Autodesk Inventor part; units mm, degrees
(part 2 of 2)
sketch "Sketch2" plane through (2, 0, 0) normal (1, 0, 0) x (0, 0, -1)
  line L0 (27.4898, 96.0981) -> (27.4898, 576.0981) projected
  line L1 (27.4898, 576.0981) -> (-362.5102, 576.0981) projected
  line L2 (-362.5102, 576.0981) -> (-362.5102, 96.0981) projected
  line L3 (-362.5102, 96.0981) -> (27.4898, 96.0981) projected
  circle A0 centre (-37.5102, 103.5981) radius 1.75 projected
  circle A1 centre (-297.5102, 568.5981) radius 1.75 projected
  circle A2 centre (-37.5102, 568.5981) radius 1.75 projected
  circle A3 centre (-355.0102, 161.0981) radius 1.75 projected
  circle A4 centre (-355.0102, 511.0981) radius 1.75 projected
  circle A5 centre (19.9898, 161.0981) radius 1.75 projected
  circle A6 centre (19.9898, 511.0981) radius 1.75 projected
  circle A7 centre (-167.5102, 568.5981) radius 1.75 projected
  circle A8 centre (-297.5102, 103.5981) radius 1.75 projected
  line L4 (7.265, 163.0981) -> (1.4915, 163.0981) projected
  line L5 (1.4915, 163.0981) -> (-1.3952, 168.0981) projected
  line L6 (-1.3952, 168.0981) -> (1.4915, 173.0981) projected
  line L7 (1.4915, 173.0981) -> (7.265, 173.0981) projected
  line L8 (7.265, 173.0981) -> (10.1518, 168.0981) projected
  line L9 (10.1518, 168.0981) -> (7.265, 163.0981) projected
  line L10 (-18.735, 143.0981) -> (-15.8482, 138.0981) projected
  line L11 (-15.8482, 138.0981) -> (-18.735, 133.0981) projected
  line L12 (-18.735, 133.0981) -> (-24.5085, 133.0981) projected
  line L13 (-24.5085, 133.0981) -> (-27.3952, 138.0981) projected
  line L14 (-27.3952, 138.0981) -> (-24.5085, 143.0981) projected
  line L15 (-24.5085, 143.0981) -> (-18.735, 143.0981) projected
  line L16 (-40.3856, 160.5981) -> (-37.4988, 165.5981) projected
  line L17 (-37.4988, 165.5981) -> (-31.7253, 165.5981) projected
  line L18 (-31.7253, 165.5981) -> (-28.8386, 160.5981) projected
  line L19 (-28.8386, 160.5981) -> (-31.7253, 155.5981) projected
  line L20 (-31.7253, 155.5981) -> (-37.4988, 155.5981) projected
  line L21 (-37.4988, 155.5981) -> (-40.3856, 160.5981) projected
  line L22 (-50.5085, 128.0981) -> (-44.735, 128.0981) projected
  line L23 (-44.735, 128.0981) -> (-41.8482, 123.0981) projected
  line L24 (-41.8482, 123.0981) -> (-44.735, 118.0981) projected
  line L25 (-44.735, 118.0981) -> (-50.5085, 118.0981) projected
  line L26 (-50.5085, 118.0981) -> (-53.3952, 123.0981) projected
  line L27 (-53.3952, 123.0981) -> (-50.5085, 128.0981) projected
  line L28 (-67.8482, 168.0981) -> (-70.735, 163.0981) projected
  line L29 (-70.735, 163.0981) -> (-76.5085, 163.0981) projected
  line L30 (-76.5085, 163.0981) -> (-79.3952, 168.0981) projected
  line L31 (-79.3952, 168.0981) -> (-76.5085, 173.0981) projected
  line L32 (-76.5085, 173.0981) -> (-70.735, 173.0981) projected
  line L33 (-70.735, 173.0981) -> (-67.8482, 168.0981) projected
  line L34 (-92.3856, 130.5981) -> (-89.4988, 135.5981) projected
  line L35 (-89.4988, 135.5981) -> (-83.7253, 135.5981) projected
  line L36 (-83.7253, 135.5981) -> (-80.8386, 130.5981) projected
  line L37 (-80.8386, 130.5981) -> (-83.7253, 125.5981) projected
  line L38 (-83.7253, 125.5981) -> (-89.4988, 125.5981) projected
  line L39 (-89.4988, 125.5981) -> (-92.3856, 130.5981) projected
  line L40 (-102.5085, 158.0981) -> (-96.735, 158.0981) projected
  line L41 (-96.735, 158.0981) -> (-93.8482, 153.0981) projected
  line L42 (-93.8482, 153.0981) -> (-96.735, 148.0981) projected
  line L43 (-96.735, 148.0981) -> (-102.5085, 148.0981) projected
  line L44 (-102.5085, 148.0981) -> (-105.3952, 153.0981) projected
  line L45 (-105.3952, 153.0981) -> (-102.5085, 158.0981) projected
  line L46 (-115.4988, 140.5981) -> (-118.3856, 145.5981) projected
  line L47 (-118.3856, 145.5981) -> (-115.4988, 150.5981) projected
  line L48 (-115.4988, 150.5981) -> (-109.7253, 150.5981) projected
  line L49 (-109.7253, 150.5981) -> (-106.8386, 145.5981) projected
  line L50 (-106.8386, 145.5981) -> (-109.7253, 140.5981) projected
  line L51 (-109.7253, 140.5981) -> (-115.4988, 140.5981) projected
  line L52 (-122.735, 143.0981) -> (-119.8482, 138.0981) projected
  line L53 (-119.8482, 138.0981) -> (-122.735, 133.0981) projected
  line L54 (-122.735, 133.0981) -> (-128.5085, 133.0981) projected
  line L55 (-128.5085, 133.0981) -> (-131.3952, 138.0981) projected
  line L56 (-131.3952, 138.0981) -> (-128.5085, 143.0981) projected
  line L57 (-128.5085, 143.0981) -> (-122.735, 143.0981) projected
  line L58 (-148.735, 143.0981) -> (-145.8482, 138.0981) projected
  line L59 (-145.8482, 138.0981) -> (-148.735, 133.0981) projected
  line L60 (-148.735, 133.0981) -> (-154.5085, 133.0981) projected
  line L61 (-154.5085, 133.0981) -> (-157.3952, 138.0981) projected
  line L62 (-157.3952, 138.0981) -> (-154.5085, 143.0981) projected
  line L63 (-154.5085, 143.0981) -> (-148.735, 143.0981) projected
  line L64 (-154.5085, 158.0981) -> (-148.735, 158.0981) projected
  line L65 (-148.735, 158.0981) -> (-145.8482, 153.0981) projected
  line L66 (-145.8482, 153.0981) -> (-148.735, 148.0981) projected
  line L67 (-148.735, 148.0981) -> (-154.5085, 148.0981) projected
  line L68 (-154.5085, 148.0981) -> (-157.3952, 153.0981) projected
  line L69 (-157.3952, 153.0981) -> (-154.5085, 158.0981) projected
  line L70 (-171.8482, 168.0981) -> (-174.735, 163.0981) projected
  line L71 (-174.735, 163.0981) -> (-180.5085, 163.0981) projected
  line L72 (-180.5085, 163.0981) -> (-183.3952, 168.0981) projected
  line L73 (-183.3952, 168.0981) -> (-180.5085, 173.0981) projected
  line L74 (-180.5085, 173.0981) -> (-174.735, 173.0981) projected
  line L75 (-174.735, 173.0981) -> (-171.8482, 168.0981) projected
  line L76 (-196.3856, 130.5981) -> (-193.4988, 135.5981) projected
  line L77 (-193.4988, 135.5981) -> (-187.7253, 135.5981) projected
  line L78 (-187.7253, 135.5981) -> (-184.8386, 130.5981) projected
  line L79 (-184.8386, 130.5981) -> (-187.7253, 125.5981) projected
  line L80 (-187.7253, 125.5981) -> (-193.4988, 125.5981) projected
  line L81 (-193.4988, 125.5981) -> (-196.3856, 130.5981) projected
  line L82 (-206.5085, 158.0981) -> (-200.735, 158.0981) projected
  line L83 (-200.735, 158.0981) -> (-197.8482, 153.0981) projected
  line L84 (-197.8482, 153.0981) -> (-200.735, 148.0981) projected
  line L85 (-200.735, 148.0981) -> (-206.5085, 148.0981) projected
  line L86 (-206.5085, 148.0981) -> (-209.3952, 153.0981) projected
  line L87 (-209.3952, 153.0981) -> (-206.5085, 158.0981) projected
  line L88 (-219.4988, 140.5981) -> (-222.3856, 145.5981) projected
  line L89 (-222.3856, 145.5981) -> (-219.4988, 150.5981) projected
  line L90 (-219.4988, 150.5981) -> (-213.7253, 150.5981) projected
  line L91 (-213.7253, 150.5981) -> (-210.8386, 145.5981) projected
  line L92 (-210.8386, 145.5981) -> (-213.7253, 140.5981) projected
  line L93 (-213.7253, 140.5981) -> (-219.4988, 140.5981) projected
  line L94 (-226.735, 143.0981) -> (-223.8482, 138.0981) projected
  line L95 (-223.8482, 138.0981) -> (-226.735, 133.0981) projected
  line L96 (-226.735, 133.0981) -> (-232.5085, 133.0981) projected
  line L97 (-232.5085, 133.0981) -> (-235.3952, 138.0981) projected
  line L98 (-235.3952, 138.0981) -> (-232.5085, 143.0981) projected
  line L99 (-232.5085, 143.0981) -> (-226.735, 143.0981) projected
  line L100 (-248.3856, 160.5981) -> (-245.4988, 165.5981) projected
  line L101 (-245.4988, 165.5981) -> (-239.7253, 165.5981) projected
  line L102 (-239.7253, 165.5981) -> (-236.8386, 160.5981) projected
  line L103 (-236.8386, 160.5981) -> (-239.7253, 155.5981) projected
  line L104 (-239.7253, 155.5981) -> (-245.4988, 155.5981) projected
  line L105 (-245.4988, 155.5981) -> (-248.3856, 160.5981) projected
  line L106 (-258.5085, 128.0981) -> (-252.735, 128.0981) projected
  line L107 (-252.735, 128.0981) -> (-249.8482, 123.0981) projected
  line L108 (-249.8482, 123.0981) -> (-252.735, 118.0981) projected
  line L109 (-252.735, 118.0981) -> (-258.5085, 118.0981) projected
  line L110 (-258.5085, 118.0981) -> (-261.3952, 123.0981) projected
  line L111 (-261.3952, 123.0981) -> (-258.5085, 128.0981) projected
  line L112 (-310.5085, 128.0981) -> (-304.735, 128.0981) projected
  line L113 (-304.735, 128.0981) -> (-301.8482, 123.0981) projected
  line L114 (-301.8482, 123.0981) -> (-304.735, 118.0981) projected
  line L115 (-304.735, 118.0981) -> (-310.5085, 118.0981) projected
  line L116 (-310.5085, 118.0981) -> (-313.3952, 123.0981) projected
  line L117 (-313.3952, 123.0981) -> (-310.5085, 128.0981) projected
  line L118 (-336.5085, 158.0981) -> (-330.735, 158.0981) projected
  line L119 (-330.735, 158.0981) -> (-327.8482, 153.0981) projected
  line L120 (-327.8482, 153.0981) -> (-330.735, 148.0981) projected
  line L121 (-330.735, 148.0981) -> (-336.5085, 148.0981) projected
  line L122 (-336.5085, 148.0981) -> (-339.3952, 153.0981) projected
  line L123 (-339.3952, 153.0981) -> (-336.5085, 158.0981) projected
  line L124 (-275.8482, 168.0981) -> (-278.735, 163.0981) projected
  line L125 (-278.735, 163.0981) -> (-284.5085, 163.0981) projected
  line L126 (-284.5085, 163.0981) -> (-287.3952, 168.0981) projected
  line L127 (-287.3952, 168.0981) -> (-284.5085, 173.0981) projected
  line L128 (-284.5085, 173.0981) -> (-278.735, 173.0981) projected
  line L129 (-278.735, 173.0981) -> (-275.8482, 168.0981) projected
  line L130 (-278.735, 143.0981) -> (-275.8482, 138.0981) projected
  line L131 (-275.8482, 138.0981) -> (-278.735, 133.0981) projected
  line L132 (-278.735, 133.0981) -> (-284.5085, 133.0981) projected
  line L133 (-284.5085, 133.0981) -> (-287.3952, 138.0981) projected
  line L134 (-287.3952, 138.0981) -> (-284.5085, 143.0981) projected
  line L135 (-284.5085, 143.0981) -> (-278.735, 143.0981) projected
  line L136 (-304.735, 143.0981) -> (-301.8482, 138.0981) projected
  line L137 (-301.8482, 138.0981) -> (-304.735, 133.0981) projected
  line L138 (-304.735, 133.0981) -> (-310.5085, 133.0981) projected
  line L139 (-310.5085, 133.0981) -> (-313.3952, 138.0981) projected
  line L140 (-313.3952, 138.0981) -> (-310.5085, 143.0981) projected
  line L141 (-310.5085, 143.0981) -> (-304.735, 143.0981) projected
  line L142 (1.4915, 128.0981) -> (7.265, 128.0981) projected
  line L143 (7.265, 128.0981) -> (10.1518, 123.0981) projected
  line L144 (10.1518, 123.0981) -> (7.265, 118.0981) projected
  line L145 (7.265, 118.0981) -> (1.4915, 118.0981) projected
  line L146 (1.4915, 118.0981) -> (-1.3952, 123.0981) projected
  line L147 (-1.3952, 123.0981) -> (1.4915, 128.0981) projected
  line L148 (-5.7253, 140.5981) -> (-11.4988, 140.5981) projected
  line L149 (-11.4988, 140.5981) -> (-14.3856, 145.5981) projected
  line L150 (-14.3856, 145.5981) -> (-11.4988, 150.5981) projected
  line L151 (-11.4988, 150.5981) -> (-5.7253, 150.5981) projected
  line L152 (-5.7253, 150.5981) -> (-2.8386, 145.5981) projected
  line L153 (-2.8386, 145.5981) -> (-5.7253, 140.5981) projected
  line L154 (-323.4988, 140.5981) -> (-326.3856, 145.5981) projected
  line L155 (-326.3856, 145.5981) -> (-323.4988, 150.5981) projected
  line L156 (-323.4988, 150.5981) -> (-317.7253, 150.5981) projected
  line L157 (-317.7253, 150.5981) -> (-314.8386, 145.5981) projected
  line L158 (-314.8386, 145.5981) -> (-317.7253, 140.5981) projected
  line L159 (-317.7253, 140.5981) -> (-323.4988, 140.5981) projected
  line L160 (-297.4988, 140.5981) -> (-300.3856, 145.5981) projected
  line L161 (-300.3856, 145.5981) -> (-297.4988, 150.5981) projected
  line L162 (-297.4988, 150.5981) -> (-291.7253, 150.5981) projected
  line L163 (-291.7253, 150.5981) -> (-288.8386, 145.5981) projected
  line L164 (-288.8386, 145.5981) -> (-291.7253, 140.5981) projected
  line L165 (-291.7253, 140.5981) -> (-297.4988, 140.5981) projected
  line L166 (-274.3856, 160.5981) -> (-271.4988, 165.5981) projected
  line L167 (-271.4988, 165.5981) -> (-265.7253, 165.5981) projected
  line L168 (-265.7253, 165.5981) -> (-262.8386, 160.5981) projected
  line L169 (-262.8386, 160.5981) -> (-265.7253, 155.5981) projected
  line L170 (-265.7253, 155.5981) -> (-271.4988, 155.5981) projected
  line L171 (-271.4988, 155.5981) -> (-274.3856, 160.5981) projected
  line L172 (-327.8482, 168.0981) -> (-330.735, 163.0981) projected
  line L173 (-330.735, 163.0981) -> (-336.5085, 163.0981) projected
  line L174 (-336.5085, 163.0981) -> (-339.3952, 168.0981) projected
  line L175 (-339.3952, 168.0981) -> (-336.5085, 173.0981) projected
  line L176 (-336.5085, 173.0981) -> (-330.735, 173.0981) projected
  line L177 (-330.735, 173.0981) -> (-327.8482, 168.0981) projected
  line L178 (-326.3856, 130.5981) -> (-323.4988, 135.5981) projected
  line L179 (-323.4988, 135.5981) -> (-317.7253, 135.5981) projected
  line L180 (-317.7253, 135.5981) -> (-314.8386, 130.5981) projected
  line L181 (-314.8386, 130.5981) -> (-317.7253, 125.5981) projected
  line L182 (-317.7253, 125.5981) -> (-323.4988, 125.5981) projected
  line L183 (-323.4988, 125.5981) -> (-326.3856, 130.5981) projected
  line L184 (-274.3856, 130.5981) -> (-271.4988, 135.5981) projected
  line L185 (-271.4988, 135.5981) -> (-265.7253, 135.5981) projected
  line L186 (-265.7253, 135.5981) -> (-262.8386, 130.5981) projected
  line L187 (-262.8386, 130.5981) -> (-265.7253, 125.5981) projected
  line L188 (-265.7253, 125.5981) -> (-271.4988, 125.5981) projected
  line L189 (-271.4988, 125.5981) -> (-274.3856, 130.5981) projected
  line L190 (-249.8482, 168.0981) -> (-252.735, 163.0981) projected
  line L191 (-252.735, 163.0981) -> (-258.5085, 163.0981) projected
  line L192 (-258.5085, 163.0981) -> (-261.3952, 168.0981) projected
  line L193 (-261.3952, 168.0981) -> (-258.5085, 173.0981) projected
  line L194 (-258.5085, 173.0981) -> (-252.735, 173.0981) projected
  line L195 (-252.735, 173.0981) -> (-249.8482, 168.0981) projected
  line L196 (-232.5085, 128.0981) -> (-226.735, 128.0981) projected
  line L197 (-226.735, 128.0981) -> (-223.8482, 123.0981) projected
  line L198 (-223.8482, 123.0981) -> (-226.735, 118.0981) projected
  line L199 (-226.735, 118.0981) -> (-232.5085, 118.0981) projected
  line L200 (-232.5085, 118.0981) -> (-235.3952, 123.0981) projected
  line L201 (-235.3952, 123.0981) -> (-232.5085, 128.0981) projected
  line L202 (-222.3856, 160.5981) -> (-219.4988, 165.5981) projected
  line L203 (-219.4988, 165.5981) -> (-213.7253, 165.5981) projected
  line L204 (-213.7253, 165.5981) -> (-210.8386, 160.5981) projected
  line L205 (-210.8386, 160.5981) -> (-213.7253, 155.5981) projected
  line L206 (-213.7253, 155.5981) -> (-219.4988, 155.5981) projected
  line L207 (-219.4988, 155.5981) -> (-222.3856, 160.5981) projected
  line L208 (-200.735, 143.0981) -> (-197.8482, 138.0981) projected
  line L209 (-197.8482, 138.0981) -> (-200.735, 133.0981) projected
  line L210 (-200.735, 133.0981) -> (-206.5085, 133.0981) projected
  line L211 (-206.5085, 133.0981) -> (-209.3952, 138.0981) projected
  line L212 (-209.3952, 138.0981) -> (-206.5085, 143.0981) projected
  line L213 (-206.5085, 143.0981) -> (-200.735, 143.0981) projected
  line L214 (-193.4988, 140.5981) -> (-196.3856, 145.5981) projected
  line L215 (-196.3856, 145.5981) -> (-193.4988, 150.5981) projected
  line L216 (-193.4988, 150.5981) -> (-187.7253, 150.5981) projected
  line L217 (-187.7253, 150.5981) -> (-184.8386, 145.5981) projected
  line L218 (-184.8386, 145.5981) -> (-187.7253, 140.5981) projected
  line L219 (-187.7253, 140.5981) -> (-193.4988, 140.5981) projected
  line L220 (-180.5085, 158.0981) -> (-174.735, 158.0981) projected
  line L221 (-174.735, 158.0981) -> (-171.8482, 153.0981) projected
  line L222 (-171.8482, 153.0981) -> (-174.735, 148.0981) projected
  line L223 (-174.735, 148.0981) -> (-180.5085, 148.0981) projected
  line L224 (-180.5085, 148.0981) -> (-183.3952, 153.0981) projected
  line L225 (-183.3952, 153.0981) -> (-180.5085, 158.0981) projected
  line L226 (-170.3856, 130.5981) -> (-167.4988, 135.5981) projected
  line L227 (-167.4988, 135.5981) -> (-161.7253, 135.5981) projected
  line L228 (-161.7253, 135.5981) -> (-158.8386, 130.5981) projected
  line L229 (-158.8386, 130.5981) -> (-161.7253, 125.5981) projected
  line L230 (-161.7253, 125.5981) -> (-167.4988, 125.5981) projected
  line L231 (-167.4988, 125.5981) -> (-170.3856, 130.5981) projected
  line L232 (-141.4988, 140.5981) -> (-144.3856, 145.5981) projected
  line L233 (-144.3856, 145.5981) -> (-141.4988, 150.5981) projected
  line L234 (-141.4988, 150.5981) -> (-135.7253, 150.5981) projected
  line L235 (-135.7253, 150.5981) -> (-132.8386, 145.5981) projected
  line L236 (-132.8386, 145.5981) -> (-135.7253, 140.5981) projected
  line L237 (-135.7253, 140.5981) -> (-141.4988, 140.5981) projected
  line L238 (-128.5085, 128.0981) -> (-122.735, 128.0981) projected
  line L239 (-122.735, 128.0981) -> (-119.8482, 123.0981) projected
  line L240 (-119.8482, 123.0981) -> (-122.735, 118.0981) projected
  line L241 (-122.735, 118.0981) -> (-128.5085, 118.0981) projected
  line L242 (-128.5085, 118.0981) -> (-131.3952, 123.0981) projected
  line L243 (-131.3952, 123.0981) -> (-128.5085, 128.0981) projected
  line L244 (-118.3856, 160.5981) -> (-115.4988, 165.5981) projected
  line L245 (-115.4988, 165.5981) -> (-109.7253, 165.5981) projected
  line L246 (-109.7253, 165.5981) -> (-106.8386, 160.5981) projected
  line L247 (-106.8386, 160.5981) -> (-109.7253, 155.5981) projected
  line L248 (-109.7253, 155.5981) -> (-115.4988, 155.5981) projected
  line L249 (-115.4988, 155.5981) -> (-118.3856, 160.5981) projected
  line L250 (-96.735, 143.0981) -> (-93.8482, 138.0981) projected
  line L251 (-93.8482, 138.0981) -> (-96.735, 133.0981) projected
  line L252 (-96.735, 133.0981) -> (-102.5085, 133.0981) projected
  line L253 (-102.5085, 133.0981) -> (-105.3952, 138.0981) projected
  line L254 (-105.3952, 138.0981) -> (-102.5085, 143.0981) projected
  line L255 (-102.5085, 143.0981) -> (-96.735, 143.0981) projected
  line L256 (-89.4988, 140.5981) -> (-92.3856, 145.5981) projected
  line L257 (-92.3856, 145.5981) -> (-89.4988, 150.5981) projected
  line L258 (-89.4988, 150.5981) -> (-83.7253, 150.5981) projected
  line L259 (-83.7253, 150.5981) -> (-80.8386, 145.5981) projected
  line L260 (-80.8386, 145.5981) -> (-83.7253, 140.5981) projected
  line L261 (-83.7253, 140.5981) -> (-89.4988, 140.5981) projected
  line L262 (-76.5085, 158.0981) -> (-70.735, 158.0981) projected
  line L263 (-70.735, 158.0981) -> (-67.8482, 153.0981) projected
  line L264 (-67.8482, 153.0981) -> (-70.735, 148.0981) projected
  line L265 (-70.735, 148.0981) -> (-76.5085, 148.0981) projected
  line L266 (-76.5085, 148.0981) -> (-79.3952, 153.0981) projected
  line L267 (-79.3952, 153.0981) -> (-76.5085, 158.0981) projected
  line L268 (-66.3856, 130.5981) -> (-63.4988, 135.5981) projected
  line L269 (-63.4988, 135.5981) -> (-57.7253, 135.5981) projected
  line L270 (-57.7253, 135.5981) -> (-54.8386, 130.5981) projected
  line L271 (-54.8386, 130.5981) -> (-57.7253, 125.5981) projected
  line L272 (-57.7253, 125.5981) -> (-63.4988, 125.5981) projected
  line L273 (-63.4988, 125.5981) -> (-66.3856, 130.5981) projected
  line L274 (-41.8482, 168.0981) -> (-44.735, 163.0981) projected
  line L275 (-44.735, 163.0981) -> (-50.5085, 163.0981) projected
  line L276 (-50.5085, 163.0981) -> (-53.3952, 168.0981) projected
  line L277 (-53.3952, 168.0981) -> (-50.5085, 173.0981) projected
  line L278 (-50.5085, 173.0981) -> (-44.735, 173.0981) projected
  line L279 (-44.735, 173.0981) -> (-41.8482, 168.0981) projected
  line L280 (-24.5085, 128.0981) -> (-18.735, 128.0981) projected
  line L281 (-18.735, 128.0981) -> (-15.8482, 123.0981) projected
  line L282 (-15.8482, 123.0981) -> (-18.735, 118.0981) projected
  line L283 (-18.735, 118.0981) -> (-24.5085, 118.0981) projected
  line L284 (-24.5085, 118.0981) -> (-27.3952, 123.0981) projected
  line L285 (-27.3952, 123.0981) -> (-24.5085, 128.0981) projected
  line L286 (-5.7253, 155.5981) -> (-11.4988, 155.5981) projected
  line L287 (-11.4988, 155.5981) -> (-14.3856, 160.5981) projected
  line L288 (-14.3856, 160.5981) -> (-11.4988, 165.5981) projected
  line L289 (-11.4988, 165.5981) -> (-5.7253, 165.5981) projected
  line L290 (-5.7253, 165.5981) -> (-2.8386, 160.5981) projected
  line L291 (-2.8386, 160.5981) -> (-5.7253, 155.5981) projected
  line L292 (-24.5085, 158.0981) -> (-18.735, 158.0981) projected
  line L293 (-18.735, 158.0981) -> (-15.8482, 153.0981) projected
  line L294 (-15.8482, 153.0981) -> (-18.735, 148.0981) projected
  line L295 (-18.735, 148.0981) -> (-24.5085, 148.0981) projected
  line L296 (-24.5085, 148.0981) -> (-27.3952, 153.0981) projected
  line L297 (-27.3952, 153.0981) -> (-24.5085, 158.0981) projected
  line L298 (-37.4988, 140.5981) -> (-40.3856, 145.5981) projected
  line L299 (-40.3856, 145.5981) -> (-37.4988, 150.5981) projected
  line L300 (-37.4988, 150.5981) -> (-31.7253, 150.5981) projected
  line L301 (-31.7253, 150.5981) -> (-28.8386, 145.5981) projected
  line L302 (-28.8386, 145.5981) -> (-31.7253, 140.5981) projected
  line L303 (-31.7253, 140.5981) -> (-37.4988, 140.5981) projected
  line L304 (-44.735, 143.0981) -> (-41.8482, 138.0981) projected
  line L305 (-41.8482, 138.0981) -> (-44.735, 133.0981) projected
  line L306 (-44.735, 133.0981) -> (-50.5085, 133.0981) projected
  line L307 (-50.5085, 133.0981) -> (-53.3952, 138.0981) projected
  line L308 (-53.3952, 138.0981) -> (-50.5085, 143.0981) projected
  line L309 (-50.5085, 143.0981) -> (-44.735, 143.0981) projected
  line L310 (-66.3856, 160.5981) -> (-63.4988, 165.5981) projected
  line L311 (-63.4988, 165.5981) -> (-57.7253, 165.5981) projected
  line L312 (-57.7253, 165.5981) -> (-54.8386, 160.5981) projected
  line L313 (-54.8386, 160.5981) -> (-57.7253, 155.5981) projected
  line L314 (-57.7253, 155.5981) -> (-63.4988, 155.5981) projected
  line L315 (-63.4988, 155.5981) -> (-66.3856, 160.5981) projected
  line L316 (-76.5085, 128.0981) -> (-70.735, 128.0981) projected
  line L317 (-70.735, 128.0981) -> (-67.8482, 123.0981) projected
  line L318 (-67.8482, 123.0981) -> (-70.735, 118.0981) projected
  line L319 (-70.735, 118.0981) -> (-76.5085, 118.0981) projected
  line L320 (-76.5085, 118.0981) -> (-79.3952, 123.0981) projected
  line L321 (-79.3952, 123.0981) -> (-76.5085, 128.0981) projected
  line L322 (-93.8482, 168.0981) -> (-96.735, 163.0981) projected
  line L323 (-96.735, 163.0981) -> (-102.5085, 163.0981) projected
  line L324 (-102.5085, 163.0981) -> (-105.3952, 168.0981) projected
  line L325 (-105.3952, 168.0981) -> (-102.5085, 173.0981) projected
  line L326 (-102.5085, 173.0981) -> (-96.735, 173.0981) projected
  line L327 (-96.735, 173.0981) -> (-93.8482, 168.0981) projected
  line L328 (-118.3856, 130.5981) -> (-115.4988, 135.5981) projected
  line L329 (-115.4988, 135.5981) -> (-109.7253, 135.5981) projected
  line L330 (-109.7253, 135.5981) -> (-106.8386, 130.5981) projected
  line L331 (-106.8386, 130.5981) -> (-109.7253, 125.5981) projected
  line L332 (-109.7253, 125.5981) -> (-115.4988, 125.5981) projected
  line L333 (-115.4988, 125.5981) -> (-118.3856, 130.5981) projected
  line L334 (-128.5085, 158.0981) -> (-122.735, 158.0981) projected
  line L335 (-122.735, 158.0981) -> (-119.8482, 153.0981) projected
  line L336 (-119.8482, 153.0981) -> (-122.735, 148.0981) projected
  line L337 (-122.735, 148.0981) -> (-128.5085, 148.0981) projected
  line L338 (-128.5085, 148.0981) -> (-131.3952, 153.0981) projected
  line L339 (-131.3952, 153.0981) -> (-128.5085, 158.0981) projected
  line L340 (-154.5085, 128.0981) -> (-148.735, 128.0981) projected
  line L341 (-148.735, 128.0981) -> (-145.8482, 123.0981) projected
  line L342 (-145.8482, 123.0981) -> (-148.735, 118.0981) projected
  line L343 (-148.735, 118.0981) -> (-154.5085, 118.0981) projected
  line L344 (-154.5085, 118.0981) -> (-157.3952, 123.0981) projected
  line L345 (-157.3952, 123.0981) -> (-154.5085, 128.0981) projected
  line L346 (-145.8482, 168.0981) -> (-148.735, 163.0981) projected
  line L347 (-148.735, 163.0981) -> (-154.5085, 163.0981) projected
  line L348 (-154.5085, 163.0981) -> (-157.3952, 168.0981) projected
  line L349 (-157.3952, 168.0981) -> (-154.5085, 173.0981) projected
  line L350 (-154.5085, 173.0981) -> (-148.735, 173.0981) projected
  line L351 (-148.735, 173.0981) -> (-145.8482, 168.0981) projected
  line L352 (-170.3856, 160.5981) -> (-167.4988, 165.5981) projected
  line L353 (-167.4988, 165.5981) -> (-161.7253, 165.5981) projected
  line L354 (-161.7253, 165.5981) -> (-158.8386, 160.5981) projected
  line L355 (-158.8386, 160.5981) -> (-161.7253, 155.5981) projected
  line L356 (-161.7253, 155.5981) -> (-167.4988, 155.5981) projected
  line L357 (-167.4988, 155.5981) -> (-170.3856, 160.5981) projected
  line L358 (-180.5085, 128.0981) -> (-174.735, 128.0981) projected
  line L359 (-174.735, 128.0981) -> (-171.8482, 123.0981) projected
  line L360 (-171.8482, 123.0981) -> (-174.735, 118.0981) projected
  line L361 (-174.735, 118.0981) -> (-180.5085, 118.0981) projected
  line L362 (-180.5085, 118.0981) -> (-183.3952, 123.0981) projected
  line L363 (-183.3952, 123.0981) -> (-180.5085, 128.0981) projected
  line L364 (-197.8482, 168.0981) -> (-200.735, 163.0981) projected
  line L365 (-200.735, 163.0981) -> (-206.5085, 163.0981) projected
  line L366 (-206.5085, 163.0981) -> (-209.3952, 168.0981) projected
  line L367 (-209.3952, 168.0981) -> (-206.5085, 173.0981) projected
  line L368 (-206.5085, 173.0981) -> (-200.735, 173.0981) projected
  line L369 (-200.735, 173.0981) -> (-197.8482, 168.0981) projected
  line L370 (-222.3856, 130.5981) -> (-219.4988, 135.5981) projected
  line L371 (-219.4988, 135.5981) -> (-213.7253, 135.5981) projected
  line L372 (-213.7253, 135.5981) -> (-210.8386, 130.5981) projected
  line L373 (-210.8386, 130.5981) -> (-213.7253, 125.5981) projected
  line L374 (-213.7253, 125.5981) -> (-219.4988, 125.5981) projected
  line L375 (-219.4988, 125.5981) -> (-222.3856, 130.5981) projected
  line L376 (-232.5085, 158.0981) -> (-226.735, 158.0981) projected
  line L377 (-226.735, 158.0981) -> (-223.8482, 153.0981) projected
  line L378 (-223.8482, 153.0981) -> (-226.735, 148.0981) projected
  line L379 (-226.735, 148.0981) -> (-232.5085, 148.0981) projected
  line L380 (-232.5085, 148.0981) -> (-235.3952, 153.0981) projected
  line L381 (-235.3952, 153.0981) -> (-232.5085, 158.0981) projected
  line L382 (-245.4988, 140.5981) -> (-248.3856, 145.5981) projected
  line L383 (-248.3856, 145.5981) -> (-245.4988, 150.5981) projected
  line L384 (-245.4988, 150.5981) -> (-239.7253, 150.5981) projected
  line L385 (-239.7253, 150.5981) -> (-236.8386, 145.5981) projected
  line L386 (-236.8386, 145.5981) -> (-239.7253, 140.5981) projected
  line L387 (-239.7253, 140.5981) -> (-245.4988, 140.5981) projected
  line L388 (-252.735, 143.0981) -> (-249.8482, 138.0981) projected
  line L389 (-249.8482, 138.0981) -> (-252.735, 133.0981) projected
  line L390 (-252.735, 133.0981) -> (-258.5085, 133.0981) projected
  line L391 (-258.5085, 133.0981) -> (-261.3952, 138.0981) projected
  line L392 (-261.3952, 138.0981) -> (-258.5085, 143.0981) projected
  line L393 (-258.5085, 143.0981) -> (-252.735, 143.0981) projected
  line L394 (-300.3856, 130.5981) -> (-297.4988, 135.5981) projected
  line L395 (-297.4988, 135.5981) -> (-291.7253, 135.5981) projected
  line L396 (-291.7253, 135.5981) -> (-288.8386, 130.5981) projected
  line L397 (-288.8386, 130.5981) -> (-291.7253, 125.5981) projected
  line L398 (-291.7253, 125.5981) -> (-297.4988, 125.5981) projected
  line L399 (-297.4988, 125.5981) -> (-300.3856, 130.5981) projected
  line L400 (-330.735, 143.0981) -> (-327.8482, 138.0981) projected
  line L401 (-327.8482, 138.0981) -> (-330.735, 133.0981) projected
  line L402 (-330.735, 133.0981) -> (-336.5085, 133.0981) projected
  line L403 (-336.5085, 133.0981) -> (-339.3952, 138.0981) projected
  line L404 (-339.3952, 138.0981) -> (-336.5085, 143.0981) projected
  line L405 (-336.5085, 143.0981) -> (-330.735, 143.0981) projected
  line L406 (-301.8482, 168.0981) -> (-304.735, 163.0981) projected
  line L407 (-304.735, 163.0981) -> (-310.5085, 163.0981) projected
  line L408 (-310.5085, 163.0981) -> (-313.3952, 168.0981) projected
  line L409 (-313.3952, 168.0981) -> (-310.5085, 173.0981) projected
  line L410 (-310.5085, 173.0981) -> (-304.735, 173.0981) projected
  line L411 (-304.735, 173.0981) -> (-301.8482, 168.0981) projected
  line L412 (-284.5085, 158.0981) -> (-278.735, 158.0981) projected
  line L413 (-278.735, 158.0981) -> (-275.8482, 153.0981) projected
  line L414 (-275.8482, 153.0981) -> (-278.735, 148.0981) projected
  line L415 (-278.735, 148.0981) -> (-284.5085, 148.0981) projected
  line L416 (-284.5085, 148.0981) -> (-287.3952, 153.0981) projected
  line L417 (-287.3952, 153.0981) -> (-284.5085, 158.0981) projected
  line L418 (-310.5085, 158.0981) -> (-304.735, 158.0981) projected
  line L419 (-304.735, 158.0981) -> (-301.8482, 153.0981) projected
  line L420 (-301.8482, 153.0981) -> (-304.735, 148.0981) projected
  line L421 (-304.735, 148.0981) -> (-310.5085, 148.0981) projected
  line L422 (-310.5085, 148.0981) -> (-313.3952, 153.0981) projected
  line L423 (-313.3952, 153.0981) -> (-310.5085, 158.0981) projected
  line L424 (7.265, 148.0981) -> (1.4915, 148.0981) projected
  line L425 (1.4915, 148.0981) -> (-1.3952, 153.0981) projected
  line L426 (-1.3952, 153.0981) -> (1.4915, 158.0981) projected
  line L427 (1.4915, 158.0981) -> (7.265, 158.0981) projected
  line L428 (7.265, 158.0981) -> (10.1518, 153.0981) projected
  line L429 (10.1518, 153.0981) -> (7.265, 148.0981) projected
  line L430 (-14.3856, 130.5981) -> (-11.4988, 135.5981) projected
  line L431 (-11.4988, 135.5981) -> (-5.7253, 135.5981) projected
  line L432 (-5.7253, 135.5981) -> (-2.8386, 130.5981) projected
  line L433 (-2.8386, 130.5981) -> (-5.7253, 125.5981) projected
  line L434 (-5.7253, 125.5981) -> (-11.4988, 125.5981) projected
  line L435 (-11.4988, 125.5981) -> (-14.3856, 130.5981) projected
  line L436 (1.4915, 143.0981) -> (7.265, 143.0981) projected
  line L437 (7.265, 143.0981) -> (10.1518, 138.0981) projected
  line L438 (10.1518, 138.0981) -> (7.265, 133.0981) projected
  line L439 (7.265, 133.0981) -> (1.4915, 133.0981) projected
  line L440 (1.4915, 133.0981) -> (-1.3952, 138.0981) projected
  line L441 (-1.3952, 138.0981) -> (1.4915, 143.0981) projected
  line L442 (-300.3856, 160.5981) -> (-297.4988, 165.5981) projected
  line L443 (-297.4988, 165.5981) -> (-291.7253, 165.5981) projected
  line L444 (-291.7253, 165.5981) -> (-288.8386, 160.5981) projected
  line L445 (-288.8386, 160.5981) -> (-291.7253, 155.5981) projected
  line L446 (-291.7253, 155.5981) -> (-297.4988, 155.5981) projected
  line L447 (-297.4988, 155.5981) -> (-300.3856, 160.5981) projected
  line L448 (-271.4988, 140.5981) -> (-274.3856, 145.5981) projected
  line L449 (-274.3856, 145.5981) -> (-271.4988, 150.5981) projected
  line L450 (-271.4988, 150.5981) -> (-265.7253, 150.5981) projected
  line L451 (-265.7253, 150.5981) -> (-262.8386, 145.5981) projected
  line L452 (-262.8386, 145.5981) -> (-265.7253, 140.5981) projected
  line L453 (-265.7253, 140.5981) -> (-271.4988, 140.5981) projected
  line L454 (-326.3856, 160.5981) -> (-323.4988, 165.5981) projected
  line L455 (-323.4988, 165.5981) -> (-317.7253, 165.5981) projected
  line L456 (-317.7253, 165.5981) -> (-314.8386, 160.5981) projected
  line L457 (-314.8386, 160.5981) -> (-317.7253, 155.5981) projected
  line L458 (-317.7253, 155.5981) -> (-323.4988, 155.5981) projected
  line L459 (-323.4988, 155.5981) -> (-326.3856, 160.5981) projected
  line L460 (-336.5085, 128.0981) -> (-330.735, 128.0981) projected
  line L461 (-330.735, 128.0981) -> (-327.8482, 123.0981) projected
  line L462 (-327.8482, 123.0981) -> (-330.735, 118.0981) projected
  line L463 (-330.735, 118.0981) -> (-336.5085, 118.0981) projected
  line L464 (-336.5085, 118.0981) -> (-339.3952, 123.0981) projected
  line L465 (-339.3952, 123.0981) -> (-336.5085, 128.0981) projected
  line L466 (-284.5085, 128.0981) -> (-278.735, 128.0981) projected
  line L467 (-278.735, 128.0981) -> (-275.8482, 123.0981) projected
  line L468 (-275.8482, 123.0981) -> (-278.735, 118.0981) projected
  line L469 (-278.735, 118.0981) -> (-284.5085, 118.0981) projected
  line L470 (-284.5085, 118.0981) -> (-287.3952, 123.0981) projected
  line L471 (-287.3952, 123.0981) -> (-284.5085, 128.0981) projected
  line L472 (-258.5085, 158.0981) -> (-252.735, 158.0981) projected
  line L473 (-252.735, 158.0981) -> (-249.8482, 153.0981) projected
  line L474 (-249.8482, 153.0981) -> (-252.735, 148.0981) projected
  line L475 (-252.735, 148.0981) -> (-258.5085, 148.0981) projected
  line L476 (-258.5085, 148.0981) -> (-261.3952, 153.0981) projected
  line L477 (-261.3952, 153.0981) -> (-258.5085, 158.0981) projected
  line L478 (-248.3856, 130.5981) -> (-245.4988, 135.5981) projected
  line L479 (-245.4988, 135.5981) -> (-239.7253, 135.5981) projected
  line L480 (-239.7253, 135.5981) -> (-236.8386, 130.5981) projected
  line L481 (-236.8386, 130.5981) -> (-239.7253, 125.5981) projected
  line L482 (-239.7253, 125.5981) -> (-245.4988, 125.5981) projected
  line L483 (-245.4988, 125.5981) -> (-248.3856, 130.5981) projected
  line L484 (-223.8482, 168.0981) -> (-226.735, 163.0981) projected
  line L485 (-226.735, 163.0981) -> (-232.5085, 163.0981) projected
  line L486 (-232.5085, 163.0981) -> (-235.3952, 168.0981) projected
  line L487 (-235.3952, 168.0981) -> (-232.5085, 173.0981) projected
  line L488 (-232.5085, 173.0981) -> (-226.735, 173.0981) projected
  line L489 (-226.735, 173.0981) -> (-223.8482, 168.0981) projected
  line L490 (-206.5085, 128.0981) -> (-200.735, 128.0981) projected
  line L491 (-200.735, 128.0981) -> (-197.8482, 123.0981) projected
  line L492 (-197.8482, 123.0981) -> (-200.735, 118.0981) projected
  line L493 (-200.735, 118.0981) -> (-206.5085, 118.0981) projected
  line L494 (-206.5085, 118.0981) -> (-209.3952, 123.0981) projected
  line L495 (-209.3952, 123.0981) -> (-206.5085, 128.0981) projected
  line L496 (-196.3856, 160.5981) -> (-193.4988, 165.5981) projected
  line L497 (-193.4988, 165.5981) -> (-187.7253, 165.5981) projected
  line L498 (-187.7253, 165.5981) -> (-184.8386, 160.5981) projected
  line L499 (-184.8386, 160.5981) -> (-187.7253, 155.5981) projected
  line L500 (-187.7253, 155.5981) -> (-193.4988, 155.5981) projected
  line L501 (-193.4988, 155.5981) -> (-196.3856, 160.5981) projected
  line L502 (-174.735, 143.0981) -> (-171.8482, 138.0981) projected
  line L503 (-171.8482, 138.0981) -> (-174.735, 133.0981) projected
  line L504 (-174.735, 133.0981) -> (-180.5085, 133.0981) projected
  line L505 (-180.5085, 133.0981) -> (-183.3952, 138.0981) projected
  line L506 (-183.3952, 138.0981) -> (-180.5085, 143.0981) projected
  line L507 (-180.5085, 143.0981) -> (-174.735, 143.0981) projected
  line L508 (-167.4988, 140.5981) -> (-170.3856, 145.5981) projected
  line L509 (-170.3856, 145.5981) -> (-167.4988, 150.5981) projected
  line L510 (-167.4988, 150.5981) -> (-161.7253, 150.5981) projected
  line L511 (-161.7253, 150.5981) -> (-158.8386, 145.5981) projected
  line L512 (-158.8386, 145.5981) -> (-161.7253, 140.5981) projected
  line L513 (-161.7253, 140.5981) -> (-167.4988, 140.5981) projected
  line L514 (-144.3856, 160.5981) -> (-141.4988, 165.5981) projected
  line L515 (-141.4988, 165.5981) -> (-135.7253, 165.5981) projected
  line L516 (-135.7253, 165.5981) -> (-132.8386, 160.5981) projected
  line L517 (-132.8386, 160.5981) -> (-135.7253, 155.5981) projected
  line L518 (-135.7253, 155.5981) -> (-141.4988, 155.5981) projected
  line L519 (-141.4988, 155.5981) -> (-144.3856, 160.5981) projected
  line L520 (-144.3856, 130.5981) -> (-141.4988, 135.5981) projected
  line L521 (-141.4988, 135.5981) -> (-135.7253, 135.5981) projected
  line L522 (-135.7253, 135.5981) -> (-132.8386, 130.5981) projected
  line L523 (-132.8386, 130.5981) -> (-135.7253, 125.5981) projected
  line L524 (-135.7253, 125.5981) -> (-141.4988, 125.5981) projected
  line L525 (-141.4988, 125.5981) -> (-144.3856, 130.5981) projected
  line L526 (-119.8482, 168.0981) -> (-122.735, 163.0981) projected
  line L527 (-122.735, 163.0981) -> (-128.5085, 163.0981) projected
  line L528 (-128.5085, 163.0981) -> (-131.3952, 168.0981) projected
  line L529 (-131.3952, 168.0981) -> (-128.5085, 173.0981) projected
  line L530 (-128.5085, 173.0981) -> (-122.735, 173.0981) projected
  line L531 (-122.735, 173.0981) -> (-119.8482, 168.0981) projected
  line L532 (-102.5085, 128.0981) -> (-96.735, 128.0981) projected
  line L533 (-96.735, 128.0981) -> (-93.8482, 123.0981) projected
  line L534 (-93.8482, 123.0981) -> (-96.735, 118.0981) projected
  line L535 (-96.735, 118.0981) -> (-102.5085, 118.0981) projected
  line L536 (-102.5085, 118.0981) -> (-105.3952, 123.0981) projected
  line L537 (-105.3952, 123.0981) -> (-102.5085, 128.0981) projected
  line L538 (-92.3856, 160.5981) -> (-89.4988, 165.5981) projected
  line L539 (-89.4988, 165.5981) -> (-83.7253, 165.5981) projected
  line L540 (-83.7253, 165.5981) -> (-80.8386, 160.5981) projected
  line L541 (-80.8386, 160.5981) -> (-83.7253, 155.5981) projected
  line L542 (-83.7253, 155.5981) -> (-89.4988, 155.5981) projected
  line L543 (-89.4988, 155.5981) -> (-92.3856, 160.5981) projected
  line L544 (-70.735, 143.0981) -> (-67.8482, 138.0981) projected
  line L545 (-67.8482, 138.0981) -> (-70.735, 133.0981) projected
  line L546 (-70.735, 133.0981) -> (-76.5085, 133.0981) projected
  line L547 (-76.5085, 133.0981) -> (-79.3952, 138.0981) projected
  line L548 (-79.3952, 138.0981) -> (-76.5085, 143.0981) projected
  line L549 (-76.5085, 143.0981) -> (-70.735, 143.0981) projected
  line L550 (-63.4988, 140.5981) -> (-66.3856, 145.5981) projected
  line L551 (-66.3856, 145.5981) -> (-63.4988, 150.5981) projected
  line L552 (-63.4988, 150.5981) -> (-57.7253, 150.5981) projected
  line L553 (-57.7253, 150.5981) -> (-54.8386, 145.5981) projected
  line L554 (-54.8386, 145.5981) -> (-57.7253, 140.5981) projected
  line L555 (-57.7253, 140.5981) -> (-63.4988, 140.5981) projected
  line L556 (-50.5085, 158.0981) -> (-44.735, 158.0981) projected
  line L557 (-44.735, 158.0981) -> (-41.8482, 153.0981) projected
  line L558 (-41.8482, 153.0981) -> (-44.735, 148.0981) projected
  line L559 (-44.735, 148.0981) -> (-50.5085, 148.0981) projected
  line L560 (-50.5085, 148.0981) -> (-53.3952, 153.0981) projected
  line L561 (-53.3952, 153.0981) -> (-50.5085, 158.0981) projected
  line L562 (-40.3856, 130.5981) -> (-37.4988, 135.5981) projected
  line L563 (-37.4988, 135.5981) -> (-31.7253, 135.5981) projected
  line L564 (-31.7253, 135.5981) -> (-28.8386, 130.5981) projected
  line L565 (-28.8386, 130.5981) -> (-31.7253, 125.5981) projected
  line L566 (-31.7253, 125.5981) -> (-37.4988, 125.5981) projected
  line L567 (-37.4988, 125.5981) -> (-40.3856, 130.5981) projected
  line L568 (-15.8482, 168.0981) -> (-18.735, 163.0981) projected
  line L569 (-18.735, 163.0981) -> (-24.5085, 163.0981) projected
  line L570 (-24.5085, 163.0981) -> (-27.3952, 168.0981) projected
  line L571 (-27.3952, 168.0981) -> (-24.5085, 173.0981) projected
  line L572 (-24.5085, 173.0981) -> (-18.735, 173.0981) projected
  line L573 (-18.735, 173.0981) -> (-15.8482, 168.0981) projected
  line L574 (-362.5102, 296.0981) -> (27.4898, 296.0981) construction
  line L575 (27.4898, 296.0981) -> (27.4898, 246.0981) construction
  line L576 (27.4898, 246.0981) -> (-362.5102, 246.0981) construction
  line L577 (-362.5102, 246.0981) -> (-362.5102, 296.0981) construction
  line L578 (-296.9111, 246.1211) -> (-303.4088, 252.6188)
  line L579 (-303.4088, 252.6188) -> (-303.4088, 296.1211)
  line L580 (-303.4088, 296.1211) -> (-285.9895, 296.1211)
  line L581 (-285.9895, 296.1211) -> (-285.9895, 246.1211)
  line L582 (-285.9895, 246.1211) -> (-296.9111, 246.1211)
  line L583 (-283.9618, 246.1211) -> (-283.9618, 260.9137)
  line L584 (-283.9618, 260.9137) -> (-251.1508, 260.9137)
  line L585 (-251.1508, 260.9137) -> (-251.1508, 246.1211)
  line L586 (-251.1508, 246.1211) -> (-283.9618, 246.1211)
  line L587 (-215.4365, 246.1672) -> (-240.3213, 246.1672)
  line L588 (-240.3213, 246.1672) -> (-248.3858, 254.2317)
  line L589 (-248.3858, 254.2317) -> (-248.3858, 282.204)
  line L590 (-248.3858, 282.204) -> (-230.736, 282.204)
  line L591 (-230.736, 282.204) -> (-230.736, 260.9598)
  line L592 (-230.736, 260.9598) -> (-215.4365, 260.9598)
  line L593 (-215.4365, 260.9598) -> (-215.4365, 246.1672)
  line L594 (-195.8512, 246.1672) -> (-213.501, 246.1672)
  line L595 (-213.501, 246.1672) -> (-213.501, 282.204)
  line L596 (-213.501, 282.204) -> (-195.8512, 282.204)
  line L597 (-195.8512, 282.204) -> (-195.8512, 246.1672)
  line L598 (-175.5286, 246.1211) -> (-186.5885, 246.1211)
  line L599 (-186.5885, 246.1211) -> (-193.0862, 252.6188)
  line L600 (-193.0862, 252.6188) -> (-193.0862, 289.6234)
  line L601 (-193.0862, 289.6234) -> (-186.5885, 296.1211)
  line L602 (-186.5885, 296.1211) -> (-175.5286, 296.1211)
  line L603 (-175.5286, 296.1211) -> (-175.5286, 246.1211)
  line L604 (-140.5517, 280.6833) -> (-173.501, 280.6833)
  line L605 (-173.501, 280.6833) -> (-173.501, 296.1211)
  line L606 (-173.501, 296.1211) -> (-140.5517, 296.1211)
  line L607 (-140.5517, 296.1211) -> (-140.5517, 280.6833)
  line L608 (-140.5517, 246.1211) -> (-173.501, 246.1211)
  line L609 (-173.501, 246.1211) -> (-173.501, 260.9137)
  line L610 (-173.501, 260.9137) -> (-140.5517, 260.9137)
  line L611 (-140.5517, 260.9137) -> (-140.5517, 246.1211)
  line L612 (-140.5517, 266.5358) -> (-173.501, 266.5358)
  line L613 (-173.501, 266.5358) -> (-173.501, 278.6557)
  line L614 (-173.501, 278.6557) -> (-140.5517, 278.6557)
  line L615 (-140.5517, 278.6557) -> (-140.5517, 266.5358)
  line L616 (-104.8374, 246.075) -> (-121.1968, 246.075)
  line L617 (-121.1968, 246.075) -> (-137.7867, 262.6649)
  line L618 (-137.7867, 262.6649) -> (-137.7867, 296.1211)
  line L619 (-137.7867, 296.1211) -> (-120.1369, 296.1211)
  line L620 (-120.1369, 296.1211) -> (-120.1369, 261.8815)
  line L621 (-120.1369, 261.8815) -> (-104.8374, 261.8815)
  line L622 (-104.8374, 261.8815) -> (-104.8374, 246.075)
  line L623 (-102.9019, 246.1211) -> (-102.9019, 296.1211)
  line L624 (-102.9019, 296.1211) -> (-85.5286, 296.1211)
  line L625 (-85.5286, 296.1211) -> (-85.5286, 262.757)
  line L626 (-85.5286, 262.757) -> (-102.9019, 246.1211)
  line L627 (-65.1139, 246.1211) -> (-76.266, 246.1211)
  line L628 (-76.266, 246.1211) -> (-82.7637, 252.6188)
  line L629 (-82.7637, 252.6188) -> (-82.7637, 289.6234)
  line L630 (-82.7637, 289.6234) -> (-76.2199, 296.1211)
  line L631 (-76.2199, 296.1211) -> (-49.8144, 296.1211)
  line L632 (-49.8144, 296.1211) -> (-49.8144, 280.6833)
  line L633 (-49.8144, 280.6833) -> (-65.1139, 280.6833)
  line L634 (-65.1139, 280.6833) -> (-65.1139, 246.1211)
  line L635 (-30.2291, 252.6649) -> (-36.7729, 246.1211)
  line L636 (-36.7729, 246.1211) -> (-63.2706, 246.1211)
  line L637 (-63.2706, 246.1211) -> (-63.2706, 260.9137)
  line L638 (-63.2706, 260.9137) -> (-47.8789, 260.9137)
  line L639 (-47.8789, 260.9137) -> (-47.8789, 296.1211)
  line L640 (-47.8789, 296.1211) -> (-36.7729, 296.1211)
  line L641 (-36.7729, 296.1211) -> (-30.2291, 289.5773)
  line L642 (-30.2291, 289.5773) -> (-30.2291, 252.6649)
  point P0 (0, 0)
  dimension "d2" = 150
  dimension "d3" = 50
  constraints: 2 vertical alignment, 2 other
  measures "d2" distance between parallel lines of L3 L576
  measures "d3" distance between parallel lines of L574 L576
extrude "Extrusion2" cut sketch "Sketch2" against normal through all contours L578 L579 L580 L581 L582 | L583 L584 L585 L586 | L587 L588 L589 L590 L591 L592 L593 | L594 L595 L596 L597 | L598 L599 L600 L601 L602 L603 | L604 L605 L606 L607 | L608 L609 L610 L611 | L612 L613 L614 L615 | L616 L617 L618 L619 L620 L621 L622 | L623 L624 L625 L626 | L627 L628 L629 L630 L631 L632 L633 L634 | L635 L636 L637 L638 L639 L640 L641 L642
body "Solid1"
